Garage Door Sensor Case (Autodesk Fusion 360 design; units mm, degrees)
Autodesk Fusion 360 part; units mm, degrees
note: some values were not read from the file. Set by a fixed rule: which sketch regions a step uses.
sketch "Sketch1" plane through (0, 0, 0) normal (0, 0, 1) x (1, 0, 0)
  line L0 (0, 0) -> (71, 0)
  line L1 (71, 0) -> (71, 52)
  line L2 (71, 52) -> (0, 52)
  line L3 (0, 52) -> (0, 0)
  circle A0 centre (14, 43) radius 3.5
  circle A1 centre (31, 44) radius 3
  line L4 (-2, 58.75) -> (73, 58.75)
  line L5 (73, 58.75) -> (73, -2)
  line L6 (73, -2) -> (-2, -2)
  line L7 (-2, -2) -> (-2, 58.75)
  line L8 (0, 52) -> (71, 52)
  line L9 (71, 52) -> (71, 54.75)
  line L10 (71, 54.75) -> (0, 54.75)
  line L11 (0, 54.75) -> (0, 52)
  line L12 (0, 54.75) -> (71, 54.75)
  line L13 (71, 54.75) -> (71, 56.75)
  line L14 (71, 56.75) -> (0, 56.75)
  line L15 (0, 56.75) -> (0, 54.75)
  line L16 (-2, -2) -> (-4, -2)
  line L17 (-4, -2) -> (-4, 58.75)
  line L18 (-4, 58.75) -> (-2, 58.75)
  line L19 (-2, 58.75) -> (-2, -2)
  line L20 (73, -2) -> (75, -2)
  line L21 (75, -2) -> (75, 58.75)
  line L22 (75, 58.75) -> (73, 58.75)
  line L23 (73, 58.75) -> (73, -2)
  dimension "d1" = 71
  dimension "d2" = 52
  dimension "d3" = 7
  dimension "d4" = 14
  dimension "d5" = 9
  dimension "d6" = 6
  dimension "d7" = 8
  dimension "d8" = 31
  dimension "d11" = 2
  dimension "d12" = 2
  dimension "d13" = 2
  dimension "d14" = 6.75
  dimension "d44" = 2.75
  dimension "d45" = 2
  dimension "d68" = 2
  dimension "d69" = 2
  constraint horizontal L0
  constraint vertical L1
  constraint horizontal L2
  constraint vertical L3
  constraint coincident L0.start L3.end
  constraint horizontal L4
  constraint vertical L5
  constraint horizontal L6
  constraint vertical L7
  constraint horizontal L8
  constraint vertical L9
  constraint horizontal L10
  constraint vertical L11
  constraint horizontal L12
  constraint vertical L13
  constraint horizontal L14
  constraint vertical L15
  constraint horizontal L16
  constraint vertical L17
  constraint horizontal L18
  constraint vertical L19
  constraint horizontal L20
  constraint vertical L21
  constraint horizontal L22
  constraint vertical L23
  measures "d1" distance of L0.start L0.end
  measures "d2" distance of L0.start L2.end
  measures "d3" diameter of A0
  measures "d4" distance of L3 A0.centre
  measures "d5" distance of L2 A0.centre
  measures "d6" diameter of A1
  measures "d7" distance of L2 A1.centre
  measures "d8" distance of L3 A1.centre
  measures "d11" distance of L1 L5
  measures "d12" distance of L0 L6
  measures "d13" distance of L3 L7
  measures "d14" distance of L2 L4
  measures "d44" distance of L2.end L10.end
  measures "d45" distance of L10.end L14.end
  measures "d62" distance of L0.start
  measures "d63" distance of L0.start
  measures "d68" distance of L6.end L16.end
  measures "d69" distance of L5.end L20.end
other "Base Mesh Feature1"
extrude "Extrude1" add sketch "Sketch1" along normal blind 2 contours L0 L1 L2 L3 L8 | L2 L8 L9 L10 L11 L12 | L10 L12 L13 L14 L15 makes body 1
ref_plane "WorkPlane1" through (71, 28.375, 1) normal (1, 0, 0) x (0, 1, 0)
extrude "Extrude2" add sketch "Sketch1" along normal blind 40 contours L4 L5 L6 L7 L19 L23 bodies 1
sketch "Sketch2" plane through (71, 26, 1) normal (1, 0, 0) x (0, 1, 0)
ref_plane "WorkPlane2" through (0, 0, 7) normal (0, 0, 1) x (1, 0, 0)
sketch "Sketch3" plane through (0, 0, 2) normal (0, 0, 1) x (-1, 0, 0)
  circle A0 centre (-14, -43) radius 3.5
  circle A1 centre (-31, -44) radius 3
  line L0 (0, -56.75) -> (0, 0)
  line L1 (0, 0) -> (-71, 0)
  line L2 (-71, 0) -> (-71, -56.75)
  line L3 (-71, 0) -> (-71, -52)
  line L4 (0, 0) -> (-71, 0)
  line L5 (-63.3, -8.3279) -> (-61, -9.6558)
  line L6 (-61, -9.6558) -> (-58.7, -8.3279)
  line L7 (-58.7, -8.3279) -> (-58.7, -5.6721)
  line L8 (-58.7, -5.6721) -> (-61, -4.3442)
  line L9 (-61, -4.3442) -> (-63.3, -5.6721)
  line L10 (-63.3, -5.6721) -> (-63.3, -8.3279)
  line L11 (-16.8, -33.8279) -> (-14.5, -35.1558)
  line L12 (-14.5, -35.1558) -> (-12.2, -33.8279)
  line L13 (-12.2, -33.8279) -> (-12.2, -31.1721)
  line L14 (-12.2, -31.1721) -> (-14.5, -29.8442)
  line L15 (-14.5, -29.8442) -> (-16.8, -31.1721)
  line L16 (-16.8, -31.1721) -> (-16.8, -33.8279)
  line L17 (0, -52) -> (0, 0)
  line L18 (-71, -52) -> (0, -52)
  line L19 (-9.5, -29.6132) -> (-14.5, -26.7265)
  line L20 (-14.5, -26.7265) -> (-19.5, -29.6132)
  line L21 (-19.5, -29.6132) -> (-19.5, -35.3868)
  line L22 (-19.5, -35.3868) -> (-14.5, -38.2735)
  line L23 (-14.5, -38.2735) -> (-9.5, -35.3868)
  line L24 (-9.5, -35.3868) -> (-9.5, -29.6132)
  line L25 (-56, -4.1132) -> (-61, -1.2265)
  line L26 (-61, -1.2265) -> (-66, -4.1132)
  line L27 (-66, -4.1132) -> (-66, -9.8868)
  line L28 (-66, -9.8868) -> (-61, -12.7735)
  line L29 (-61, -12.7735) -> (-56, -9.8868)
  line L30 (-56, -9.8868) -> (-56, -4.1132)
  line L31 (0, -52) -> (-3.5, -52)
  line L32 (-3.5, -52) -> (-3.5, 0)
  line L33 (-3.5, 0) -> (0, 0)
  line L34 (0, 0) -> (0, -52)
  line L35 (-71, -52) -> (-67.5, -52)
  line L36 (-67.5, -52) -> (-67.5, 0)
  line L37 (-67.5, 0) -> (-71, 0)
  line L38 (-71, 0) -> (-71, -52)
  line L39 (0, 0) -> (-71, 0)
  line L40 (-71, 0) -> (-71, -2.8)
  line L41 (-71, -2.8) -> (0, -2.8)
  line L42 (0, -2.8) -> (0, 0)
  line L43 (-71, -56.75) -> (0, -56.75)
  point P0 (-32.363, -13.2997)
  point P1 (-61, -7)
  point P2 (-14.5, -32.5)
  point P3 (-14.5, -32.5)
  point P4 (-61, -7)
  dimension "d23" = 2.3
  dimension "d24" = 10
  dimension "d25" = 7
  dimension "d26" = 2.3
  dimension "d27" = 14.5
  dimension "d28" = 19.5
  dimension "d29" = 5
  dimension "d30" = 5
  dimension "d35" = 3.5
  dimension "d36" = 3.5
  dimension "d37" = 2.8
  constraint coincident P3 P2
  constraint coincident P4 P1
  constraint horizontal L31
  constraint vertical L32
  constraint horizontal L33
  constraint vertical L34
  constraint coincident L17.start L18.end
  constraint horizontal L35
  constraint vertical L36
  constraint horizontal L37
  constraint vertical L38
  constraint coincident L3.end L18.start
  constraint coincident L1.end L2.start
  constraint coincident L0.end L1.start
  constraint horizontal L39
  constraint vertical L40
  constraint horizontal L41
  constraint vertical L42
  measures "d23" distance of P4 L10
  measures "d24" distance of L3 P4
  measures "d25" distance of L4 P4
  measures "d26" distance of P3 L16
  measures "d27" distance of P3 L17
  measures "d28" distance of P3 L18
  measures "d29" distance of P3 L24
  measures "d30" distance of P4 L30
  measures "d35" distance of L17.start L31.end
  measures "d36" distance of L3.end L35.end
  measures "d37" distance of L0.end L41.end
extrude "Extrude3" add sketch "Sketch3" along normal blind 3 contours L25 L26 L41 | L25 L26 L27 L28 L29 L30 L41 | L5 L6 L7 L8 L9 L10 | L11 L12 L13 L14 L15 L16 | L19 L20 L21 L22 L23 L24 bodies 1
extrude "Extrude4" add sketch "Sketch3" along normal blind 5 contours L25 L26 L41 | L25 L26 L27 L28 L29 L30 L41 | L19 L20 L21 L22 L23 L24 bodies 1
extrude "Extrude5" add sketch "Sketch3" along normal blind 5 contours L0 L17 L18 L31 L32 L34 L41 | L0 L1 L4 L17 L32 L33 L34 L39 L41 L42 | L2 L3 L18 L35 L36 L38 L41 | L1 L4 L25 L26 L32 L36 L39 L41 | L1 L2 L3 L4 L36 L37 L38 L39 L40 L41 | L25 L26 L41 bodies 1
ref_plane "WorkPlane3" through (35.5, 26, 7) normal (0, 0, 1) x (1, 0, 0)
ref_plane "WorkPlane4" through (35.5, 61.5, 20) normal (0, 1, 0) x (-1, 0, 0)
extrude "Extrude6" add sketch "Sketch3" along normal blind 11 contours L0 L2 L18 L31 L35 L43 bodies 1
sketch "Sketch4" plane through (0, 0, 0) normal (0, 1, 0) x (1, 0, 0)
  line L0 (44, -12.5) -> (36, -12.5)
  line L1 (36, -12.5) -> (36, -7)
  line L2 (36, -7) -> (44, -7)
  line L3 (44, -7) -> (44, -12.5)
  line L4 (73, 0) -> (-2, 0)
  line L5 (71, -7) -> (71, -40)
  line L6 (13, -27) -> (24, -27)
  line L7 (24, -27) -> (24, -21)
  line L8 (24, -21) -> (13, -21)
  line L9 (13, -21) -> (13, -27)
  line L10 (-2, 0) -> (-2, -40)
  point P0 (71, -2)
  dimension "d48" = 5.5
  dimension "d49" = 8
  dimension "d55" = 7
  dimension "d59" = 27
  dimension "d60" = 21
  dimension "d61" = 15
  dimension "d62" = 11
  dimension "d63" = 6
  constraint horizontal L0
  constraint vertical L1
  constraint horizontal L2
  constraint vertical L3
  constraint horizontal L6
  constraint vertical L7
  constraint horizontal L8
  constraint vertical L9
  measures "d48" distance of L0.start L2.end
  measures "d49" distance of L1.end L2.end
  measures "d55" distance of L2 L4
  measures "d59" distance of L2.end L5
  measures "d60" distance of L4 L8
  measures "d61" distance of L9 L10
  measures "d62" distance of L6.start L6.end
  measures "d63" distance of L6.end L7.end
ref_plane "WorkPlane5" through (35.5, 27.4, 2) normal (0, 0, 1) x (-1, 0, 0)
extrude "Extrude8" cut sketch "Sketch4" against normal blind 6 bodies 1
sketch "Sketch6" plane through (0, 0, 0) normal (0, 1, 0) x (1, 0, 0)
  line L0 (59.9269, -24) -> (47.9269, -24)
  line L1 (47.9269, -24) -> (47.9269, -16)
  line L2 (47.9269, -16) -> (59.9269, -16)
  line L3 (59.9269, -16) -> (59.9269, -24)
  line L4 (-2, 0) -> (73, 0)
  dimension "d64" = 12
  dimension "d65" = 8
  dimension "d96" = 16
  constraint horizontal L0
  constraint vertical L1
  constraint horizontal L2
  constraint vertical L3
  measures "d64" distance of L0.start L0.end
  measures "d65" distance of L0.end L1.end
  measures "d96" distance of L2 L4
sketch "Sketch5" plane through (0, 0, 0) normal (0, 1, 0) x (1, 0, 0)
  line L0 (50.8557, -4.5386) -> (42.8557, -4.5386)
  line L1 (42.8557, -4.5386) -> (42.8557, -9.5386)
  line L2 (42.8557, -9.5386) -> (50.8557, -9.5386)
  line L3 (50.8557, -9.5386) -> (50.8557, -4.5386)
  dimension "d52" = 8
  dimension "d53" = 5
  constraint horizontal L0
  constraint vertical L1
  constraint horizontal L2
  constraint vertical L3
  measures "d52" distance of L0.start L0.end
  measures "d53" distance of L0.start L2.end
extrude "Extrude9" cut sketch "Sketch6" along normal blind 77 bodies 1
extrude "Extrude10" add sketch "Sketch1" along normal blind 1.5 from surface at 38.5 contours L7 L16 L17 L18 L19 | L5 L20 L21 L22 L23 bodies 1
sketch "Sketch8" plane through (0, 0, 40) normal (0, 0, 1) x (-1, 0, 0)
  line L0 (0, 0) -> (0, -56.75)
  line L1 (0, -56.75) -> (-71, -56.75)
  line L2 (-71, -56.75) -> (-71, 0)
  line L3 (-71, 0) -> (0, 0)
  circle A0 centre (-15, -43.75) radius 3
  circle A1 centre (-56, -43.75) radius 3
  line L4 (0, -56.75) -> (-71, -56.75)
  line L5 (-71, -56.75) -> (-71, 0)
  line L6 (-71, 0) -> (0, 0)
  line L7 (0, 0) -> (0, -56.75)
  line L8 (6.5, -58.75) -> (-77.5, -58.75)
  line L9 (-77.5, -58.75) -> (-77.5, 4)
  line L10 (-77.5, 4) -> (6.5, 4)
  line L11 (6.5, 4) -> (6.5, -58.75)
  line L12 (6.5, -58.75) -> (4.5, -58.75)
  line L13 (4.5, -58.75) -> (4.5, 4)
  line L14 (4.5, 4) -> (6.5, 4)
  line L15 (6.5, 4) -> (6.5, -58.75)
  line L16 (-77.5, -58.75) -> (-75.5, -58.75)
  line L17 (-75.5, -58.75) -> (-75.5, 4)
  line L18 (-75.5, 4) -> (-77.5, 4)
  line L19 (-77.5, 4) -> (-77.5, -58.75)
  line L20 (6.5, 4) -> (2.5, 4)
  line L21 (2.5, 4) -> (2.5, -58.75)
  line L22 (2.5, -58.75) -> (6.5, -58.75)
  line L23 (6.5, -58.75) -> (6.5, 4)
  line L24 (-77.5, -58.75) -> (-73.5, -58.75)
  line L25 (-73.5, -58.75) -> (-73.5, 4)
  line L26 (-73.5, 4) -> (-77.5, 4)
  line L27 (-77.5, 4) -> (-77.5, -58.75)
  line L28 (6.5, 4) -> (-78, 4)
  line L29 (-78, 4) -> (-78, 2)
  line L30 (-78, 2) -> (6.5, 2)
  line L31 (6.5, 2) -> (6.5, 4)
  dimension "d85" = 6
  dimension "d86" = 6
  dimension "d87" = 13
  dimension "d88" = 13
  dimension "d89" = 15
  dimension "d90" = 15
  dimension "d97" = 4
  dimension "d98" = 6.5
  dimension "d99" = 6.5
  dimension "d100" = 2
  dimension "d101" = 2
  dimension "d102" = 2
  dimension "d103" = 4
  dimension "d104" = 4
  dimension "d105" = 2
  constraint horizontal L4
  constraint vertical L5
  constraint horizontal L6
  constraint vertical L7
  constraint coincident L2.end L3.start
  constraint coincident L0.end L1.start
  constraint horizontal L8
  constraint vertical L9
  constraint horizontal L10
  constraint vertical L11
  constraint horizontal L12
  constraint vertical L13
  constraint horizontal L14
  constraint vertical L15
  constraint coincident L10 L13.end
  constraint horizontal L16
  constraint vertical L17
  constraint horizontal L18
  constraint vertical L19
  constraint horizontal L20
  constraint vertical L21
  constraint horizontal L22
  constraint vertical L23
  constraint horizontal L24
  constraint vertical L25
  constraint horizontal L26
  constraint vertical L27
  constraint horizontal L28
  constraint vertical L29
  constraint horizontal L30
  constraint vertical L31
  measures "d85" diameter of A0
  measures "d86" diameter of A1
  measures "d87" distance of L1 A1.centre
  measures "d88" distance of L1 A0.centre
  measures "d89" distance of L2 A1.centre
  measures "d90" distance of L0 A0.centre
  measures "d97" distance of L6 L10
  measures "d98" distance of L5 L9
  measures "d99" distance of L7 L11
  measures "d100" distance of L4 L8
  measures "d101" distance of L13 L15
  measures "d102" distance of L8.end L16.end
  measures "d103" distance of L10.end L20.end
  measures "d104" distance of L8.end L24.end
  measures "d105" distance of L10.end L30.end
extrude "Extrude11" add sketch "Sketch8" along normal blind 2 separate body contours L0 L1 L2 L3 L4 L5 L6 L7 | L8 L11 L12 L13 L15 L22 L23 L30 | L8 L13 L21 L22 L30 | L10 L11 L13 L14 L15 L20 L23 L28 L30 L31 | L8 L21 L25 L30 | L10 L13 L20 L21 L28 L30 | L8 L17 L24 L25 L30 | L10 L21 L25 L28 L30 | L8 L9 L16 L17 L19 L24 L27 L30 | L10 L17 L25 L26 L28 L30 | L9 L10 L17 L18 L19 L26 L27 L28 L30 makes body 2
extrude "Extrude12" add sketch "Sketch8" against normal blind 5 contours L8 L11 L12 L13 L15 L22 L23 L30 | L10 L11 L13 L14 L15 L20 L23 L28 L30 L31 | L10 L13 L20 L21 L28 L30 | L10 L21 L25 L28 L30 | L8 L9 L16 L17 L19 L24 L27 L30 | L10 L17 L25 L26 L28 L30 | L9 L10 L17 L18 L19 L26 L27 L28 L30 bodies 2
extrude "Extrude13" add sketch "Sketch8" against normal blind 2 from surface at -3 contours L8 L13 L21 L22 L30 | L8 L17 L24 L25 L30 bodies 2
fillet "Fillet1" radius 1.5 8 edges at (73, -2, 19.25) (35.5, -2, 0) (73, 28.375, 0) (-2, -2, 19.25) (-2, 28.375, 0) (35.5, 58.75, 0) (73, 58.75, 19.25) (-2, 58.75, 19.25) on bodies 1
fillet "Fillet2" radius 2 4 edges at (59.9269, 57.75, 24) (47.9269, 57.75, 16) (47.9269, 57.75, 24) (59.9269, 57.75, 16) on bodies 1
fillet "Fillet3" radius 1.5 4 edges at (13, -1, 27) (13, -1, 21) (24, -1, 27) (24, -1, 21) on bodies 1
